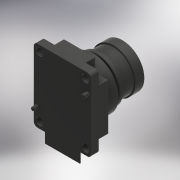
# Autodesk Inventor part: xtion_ir_cam
Saved by Autodesk Inventor 2017 (Build 210142000, 142)
## iProperties
Created: 2016-11-18
Part Number: xtion_ir_cam
Material: Thermoplastic Resin
Document SubType Name: Modeling
Designer: Ali
Density: 1.28 g/cm^3
Appearance: Smooth - Black
Author: Ali
Autodesk Inventor part; units mm, degrees
ref_plane "YZ Plane" through (0, 0, 0) normal (1, 0, 0) x (0, 1, 0)
ref_plane "XZ Plane" through (0, 0, 0) normal (0, 1, 0) x (-1, 0, 0)
ref_plane "XY Plane" through (0, 0, 0) normal (0, 0, 1) x (1, 0, 0)
sketch "Sketch1" plane through (0, 0, 0) normal (0, 1, 0) x (-1, 0, 0)
  line L0 (-7.875, 9.975) -> (7.875, 9.975)
  line L1 (7.875, 9.975) -> (7.875, -9.975)
  line L2 (7.875, -9.975) -> (-7.875, -9.975)
  line L3 (-7.875, -9.975) -> (-7.875, 9.975)
  line L4 (-7.875, 9.975) -> (7.875, -9.975) construction
  line L5 (7.875, 9.975) -> (-7.875, -9.975) construction
  point P0 (0, 0)
  dimension "d0" = 15.75
  dimension "d1" = 19.95
  constraints: 12 end point, 2 midpoint, 2 parallel, 1 horizontal, 1 perpendicular
  measures "d0" distance of L1.end L2.end
  measures "d1" distance of L0.end L1.end
extrude "Extrusion1" add sketch "Sketch1" along normal blind 4.7
sketch "Sketch2" plane through (0, 4.7, 0) normal (0, 1, 0) x (1, 0, 0)
  line L0 (-7.875, -9.975) -> (7.875, -9.975) projected
  line L1 (7.875, -9.975) -> (7.875, 9.975) projected
  line L2 (7.875, 9.975) -> (-7.875, 9.975) projected
  line L3 (-7.875, 9.975) -> (-7.875, -9.975) projected
  line L4 (-7.875, 9.975) -> (-7.875, -9.975) projected
  line L5 (-7.875, 9.975) -> (-4.275, 9.975)
  line L6 (-4.275, 9.975) -> (-4.275, 7.875)
  line L7 (-5.775, 6.375) -> (-7.875, 6.375)
  line L8 (-7.875, 6.375) -> (-7.875, 9.975)
  arc A0 (-5.775, 6.375) -> (-4.275, 7.875) centre (-5.775, 7.875) ccw
  line L9 (0, 0) -> (-2.9441, 0)
  line L10 (0, 0) -> (0, 2.9441)
  line L11 (-4.275, -9.975) -> (-4.275, -7.875)
  line L12 (-5.775, -6.375) -> (-7.875, -6.375)
  arc A1 (-4.275, -7.875) -> (-5.775, -6.375) centre (-5.775, -7.875) ccw
  line L13 (4.275, 9.975) -> (4.275, 7.875)
  line L14 (5.775, 6.375) -> (7.875, 6.375)
  arc A2 (4.275, 7.875) -> (5.775, 6.375) centre (5.775, 7.875) ccw
  line L15 (5.775, -6.375) -> (7.875, -6.375)
  arc A3 (5.775, -6.375) -> (4.275, -7.875) centre (5.775, -7.875) ccw
  line L16 (4.275, -9.975) -> (4.275, -7.875)
  line L17 (-7.875, -9.975) -> (7.875, -9.975) projected
  line L18 (-4.275, -9.975) -> (-7.875, -9.975)
  line L19 (-7.875, -9.975) -> (-7.875, -6.375)
  line L20 (4.275, -9.975) -> (7.875, -9.975)
  line L21 (4.275, -9.975) -> (7.875, -9.975)
  line L22 (7.875, -9.975) -> (7.875, 9.975) projected
  line L23 (7.875, 6.375) -> (7.875, 9.975)
  line L24 (7.875, 9.975) -> (4.275, 9.975)
  line L25 (7.875, 9.975) -> (-7.875, 9.975) projected
  line L26 (7.875, -9.975) -> (7.875, -6.375)
  point P0 (-4.275, 6.375)
  dimension "d4" = 3.6
  dimension "d5" = 3.6
  dimension "d6" = 1.5
  constraints: 38 end point, 15 symmetric about line, 8 point on circle, 5 collinear, 4 centre point, 3 horizontal, 2 parallel, 2 perpendicular, 2 point on line, 2 tangent, 1 vertical, 3 other
  measures "d4" distance of point (-4.275, 6.375) L7.end
  measures "d5" distance of L5.end point (-4.275, 6.375)
  measures "d6" radius of A0
extrude "Extrusion2" cut sketch "Sketch2" against normal blind 2.6 contours L3 L12 A1 L11 L0 | L16 A3 L15 L1 L0 | L3 L2 L6 A0 L7 | L14 A2 L13 L2 L1
sketch "Sketch3" plane through (0, 0, 0) normal (1, 0, 0) x (0, 1, 0)
  line L0 (2.1, -6.375) -> (4.7, -6.375) projected
  line L1 (4.7, 6.375) -> (4.7, -6.375) projected
  line L2 (4.7, 6.375) -> (2.1, 6.375) projected
  line L3 (2.1, 6.375) -> (2.1, 9.975) projected
  line L4 (0, 9.975) -> (2.1, 9.975) projected
  line L5 (0, -9.975) -> (0, 9.975) projected
  line L6 (0, -9.975) -> (2.1, -9.975) projected
  line L7 (2.1, -9.975) -> (2.1, -6.375) projected
  line L8 (4.7, 0) -> (22.768, 0)
  line L9 (4.7, 6.375) -> (4.7, -6.375) projected
  line L10 (4.7, -7) -> (8.4, -7)
  line L11 (8.4, -7) -> (8.4, -5.65)
  line L12 (8.4, -5.65) -> (9.4, -5.65)
  line L13 (9.4, -5.65) -> (9.4, -6.28)
  line L14 (9.4, -6.28) -> (10.4, -6.28)
  line L15 (10.4, -6.28) -> (10.4, -5.65)
  line L16 (10.4, -5.65) -> (14, -5.65)
  line L17 (14, -5.65) -> (14, -6)
  line L18 (14, -6) -> (16.5, -6)
  line L19 (16.5, -6) -> (16.5, -3.48)
  line L20 (14.7, 0) -> (4.7, 0)
  line L21 (4.7, 0) -> (4.7, -7)
  line L22 (16.5, -3.48) -> (14.7, -2.8)
  line L23 (14.7, -2.8) -> (14.7, 0)
  arc A0 (14.7, -2.8) -> (16.1269, 0) centre (12.6664, 0) ccw
  line L24 (16.1269, 0) -> (14.7, 0)
  point P0 (0, 0)
  point P1 (16.5, 0)
  dimension "d9" = 14
  dimension "d10" = 11.3
  dimension "d11" = 12.56
  dimension "d12" = 12
  dimension "d13" = 16.5
  dimension "d14" = 2.5
  dimension "d15" = 3.7
  dimension "d16" = 1
  dimension "d17" = 1
  dimension "d18" = 3.6
  dimension "d20" = 6.96
  dimension "d21" = 5.6
  dimension "d22" = 1.8
  constraints: 32 end point, 10 perpendicular, 6 point on line, 2 horizontal, 2 point on circle, 1 centre point, 1 collinear, 1 midpoint, 1 vertical
  measures "d9" diameter of L10 L8
  measures "d10" diameter of L12 L8
  measures "d11" diameter of L14 L8
  measures "d12" diameter of L18 L8
  measures "d13" distance between parallel lines of L5 L19
  measures "d14" distance of L17.end L18.end
  measures "d15" distance of L10.start L10.end
  measures "d16" distance of L11.end L12.end
  measures "d17" distance of L13.end L14.end
  measures "d18" distance of L15.end L16.end
  measures "d20" diameter of L19.end L8
  measures "d21" diameter of L22.end L8
  measures "d22" distance between parallel lines of L23 L19
revolve "Revolution1" add sketch "Sketch3" angle 360 about axis through (0, 4.7, 0) along (0, 1, 0) contours L1 L8 L23 L22 L19 L18 L17 L16 L15 L14 L13 L12 L11 L10 L21 | L8 A0 L23
sketch "Sketch4" plane through (0, 2.1, 0) normal (0, 1, 0) x (1, 0, 0)
  line L0 (7.875, -9.975) -> (-7.875, -9.975) projected
  line L1 (-7.875, -9.975) -> (-7.875, 9.975) projected
  line L2 (-7.875, 9.975) -> (7.875, 9.975) projected
  line L3 (7.875, 9.975) -> (7.875, -9.975) projected
  line L4 (6.3, -8.25) -> (-6.3, -8.25)
  line L5 (-6.3, -8.25) -> (-6.3, 8.25)
  line L6 (-6.3, 8.25) -> (6.3, 8.25)
  line L7 (6.3, 8.25) -> (6.3, -8.25)
  line L8 (6.3, -8.25) -> (-6.3, 8.25) construction
  line L9 (-6.3, -8.25) -> (6.3, 8.25) construction
  point P0 (0, 0)
  dimension "d23" = 12.6
  dimension "d24" = 16.5
  constraints: 12 end point, 4 coincident, 2 midpoint, 2 parallel, 1 horizontal, 1 perpendicular
  measures "d23" distance of L5.end L6.end
  measures "d24" distance of L6.end L4.start
hole "Hole1" at (-6.3, 2.1, 8.25) at (6.3, 2.1, 8.25) at (6.3, 2.1, -8.25) at (-6.3, 2.1, -8.25) direction (0, -1, 0) diameter 2 end through all
sketch "Sketch5" plane through (0, 0, 0) normal (0, -1, 0) x (1, 0, 0)
  circle A0 centre (6.95, 5) radius 0.5
  circle A1 centre (-6.95, -5) radius 0.5
  line L0 (6.95, 5) -> (-6.95, -5) construction
  point P0 (0, 0)
  point P1 (0, 0)
  dimension "d32" = 1
  dimension "d33" = 1
  dimension "d34" = 13.9
  dimension "d35" = 10
  constraints: 2 centre point, 2 end point, 1 coincident, 1 midpoint
  measures "d32" diameter of A0
  measures "d33" diameter of A1
  measures "d34" horizontal distance of L0.end L0.start
  measures "d35" vertical distance of L0.start L0.end
extrude "Extrusion3" add sketch "Sketch5" along normal blind 1.36
fillet "Fillet1" radius 0.3 2 edges at (6.45, -1.36, 5) (-7.45, -1.36, -5)
fillet "Fillet2" radius 1 4 edges at (-7.875, 1.05, 9.975) (7.875, 1.05, 9.975) (7.875, 1.05, -9.975) (-7.875, 1.05, -9.975)
sketch "Sketch6" plane through (4.275, 4.7, -9.975) normal (0, 0, -1) x (-1, 0, 0)
  line L0 (-0.525, -4.5) -> (9.075, -4.5)
  line L1 (9.075, -4.5) -> (9.075, -4.7)
  line L2 (9.075, -4.7) -> (-0.525, -4.7)
  line L3 (-0.525, -4.7) -> (-0.525, -4.5)
  line L4 (-0.525, -4.5) -> (9.075, -4.7) construction
  line L5 (9.075, -4.5) -> (-0.525, -4.7) construction
  line L6 (11.15, -4.7) -> (-2.6, -4.7) projected
  line L7 (4.275, -4.7) -> (4.275, -1.2739) construction
  point P0 (4.275, -4.7)
  point P1 (4.275, -4.6)
  point P2 (4.275, -4.6)
  dimension "d40" = 0.2
  dimension "d41" = 9.6
  constraints: 14 end point, 5 midpoint, 2 parallel, 1 horizontal, 1 perpendicular, 1 point on line, 1 vertical
  measures "d40" distance of L0.end L1.end
  measures "d41" distance of L0.start L0.end
extrude "Extrusion4" add sketch "Sketch6" along normal blind 2.75
body "Solid1"
